Autodesk Fusion 360 part; units mm, degrees
(part 3 of 4)
sketch "Sketch3" plane through (0, 1.5, 0) normal (0, 1, 0) x (-1, 0, 0)
  arc A0 (-294.5875, 3) -> (-291.5875, 0) centre (-291.5875, 3) ccw
  line L0 (-291.5875, 0) -> (-3, 0)
  arc A1 (-3, 0) -> (0, 3) centre (-3, 3) ccw
  line L1 (0, 3) -> (0, 137)
  arc A2 (0, 137) -> (-3, 140) centre (-3, 137) ccw
  line L2 (-3, 140) -> (-327, 140)
  arc A3 (-327, 140) -> (-330, 137) centre (-327, 137) ccw
  line L3 (-330, 137) -> (-330, 70.475)
  arc A4 (-330, 70.475) -> (-327, 67.475) centre (-327, 70.475) ccw
  line L4 (-327, 67.475) -> (-297.5875, 67.475)
  arc A5 (-294.5875, 64.475) -> (-297.5875, 67.475) centre (-297.5875, 64.475) ccw
  line L5 (-294.5875, 64.475) -> (-294.5875, 3)
  arc A6 (-96.5875, 53.475) -> (-96.0875, 53.975) centre (-96.5875, 53.975) ccw
  line L6 (-96.5875, 53.475) -> (-109.5875, 53.475)
  arc A7 (-110.0875, 53.975) -> (-109.5875, 53.475) centre (-109.5875, 53.975) ccw
  line L7 (-110.0875, 53.975) -> (-110.0875, 66.975)
  arc A8 (-109.5875, 67.475) -> (-110.0875, 66.975) centre (-109.5875, 66.975) ccw
  line L8 (-109.5875, 67.475) -> (-96.5875, 67.475)
  arc A9 (-96.0875, 66.975) -> (-96.5875, 67.475) centre (-96.5875, 66.975) ccw
  line L9 (-96.0875, 66.975) -> (-96.0875, 53.975)
  line L10 (-105.6125, 24.1125) -> (-105.6125, 11.1125)
  arc A10 (-106.1125, 10.6125) -> (-105.6125, 11.1125) centre (-106.1125, 11.1125) ccw
  line L11 (-106.1125, 10.6125) -> (-119.1125, 10.6125)
  arc A11 (-119.6125, 11.1125) -> (-119.1125, 10.6125) centre (-119.1125, 11.1125) ccw
  line L12 (-119.6125, 11.1125) -> (-119.6125, 24.1125)
  arc A12 (-119.1125, 24.6125) -> (-119.6125, 24.1125) centre (-119.1125, 24.1125) ccw
  line L13 (-119.1125, 24.6125) -> (-106.1125, 24.6125)
  arc A13 (-105.6125, 24.1125) -> (-106.1125, 24.6125) centre (-106.1125, 24.1125) ccw
  arc A14 (-201.3625, 34.425) -> (-200.8625, 34.925) centre (-201.3625, 34.925) ccw
  line L14 (-201.3625, 34.425) -> (-214.3625, 34.425)
  arc A15 (-214.8625, 34.925) -> (-214.3625, 34.425) centre (-214.3625, 34.925) ccw
  line L15 (-214.8625, 34.925) -> (-214.8625, 47.925)
  arc A16 (-214.3625, 48.425) -> (-214.8625, 47.925) centre (-214.3625, 47.925) ccw
  line L16 (-214.3625, 48.425) -> (-201.3625, 48.425)
  arc A17 (-200.8625, 47.925) -> (-201.3625, 48.425) centre (-201.3625, 47.925) ccw
  line L17 (-200.8625, 47.925) -> (-200.8625, 34.925)
  arc A18 (-53.725, 91.575) -> (-53.225, 92.075) centre (-53.725, 92.075) ccw
  line L18 (-53.725, 91.575) -> (-66.725, 91.575)
  arc A19 (-67.225, 92.075) -> (-66.725, 91.575) centre (-66.725, 92.075) ccw
  line L19 (-67.225, 92.075) -> (-67.225, 105.075)
  arc A20 (-66.725, 105.575) -> (-67.225, 105.075) centre (-66.725, 105.075) ccw
  line L20 (-66.725, 105.575) -> (-53.725, 105.575)
  arc A21 (-53.225, 105.075) -> (-53.725, 105.575) centre (-53.725, 105.075) ccw
  line L21 (-53.225, 105.075) -> (-53.225, 92.075)
  arc A22 (-220.4125, 34.425) -> (-219.9125, 34.925) centre (-220.4125, 34.925) ccw
  line L22 (-220.4125, 34.425) -> (-233.4125, 34.425)
  arc A23 (-233.9125, 34.925) -> (-233.4125, 34.425) centre (-233.4125, 34.925) ccw
  line L23 (-233.9125, 34.925) -> (-233.9125, 47.925)
  arc A24 (-233.4125, 48.425) -> (-233.9125, 47.925) centre (-233.4125, 47.925) ccw
  line L24 (-233.4125, 48.425) -> (-220.4125, 48.425)
  arc A25 (-219.9125, 47.925) -> (-220.4125, 48.425) centre (-220.4125, 47.925) ccw
  line L25 (-219.9125, 47.925) -> (-219.9125, 34.925)
  arc A26 (-283.4755, 35.425) -> (-282.9755, 35.925) centre (-283.4755, 35.925) ccw
  line L26 (-283.4755, 35.425) -> (-289.4755, 35.425)
  arc A27 (-289.9755, 35.925) -> (-289.4755, 35.425) centre (-289.4755, 35.925) ccw
  line L27 (-289.9755, 35.925) -> (-289.9755, 49.925)
  arc A28 (-289.4755, 50.425) -> (-289.9755, 49.925) centre (-289.4755, 49.925) ccw
  line L28 (-289.4755, 50.425) -> (-283.4755, 50.425)
  arc A29 (-282.9755, 49.925) -> (-283.4755, 50.425) centre (-283.4755, 49.925) ccw
  line L29 (-282.9755, 49.925) -> (-282.9755, 35.925)
  arc A30 (-101.35, 72.525) -> (-100.85, 73.025) centre (-101.35, 73.025) ccw
  line L30 (-101.35, 72.525) -> (-114.35, 72.525)
  arc A31 (-114.85, 73.025) -> (-114.35, 72.525) centre (-114.35, 73.025) ccw
  line L31 (-114.85, 73.025) -> (-114.85, 86.025)
  arc A32 (-114.35, 86.525) -> (-114.85, 86.025) centre (-114.35, 86.025) ccw
  line L32 (-114.35, 86.525) -> (-101.35, 86.525)
  arc A33 (-100.85, 86.025) -> (-101.35, 86.525) centre (-101.35, 86.025) ccw
  line L33 (-100.85, 86.025) -> (-100.85, 73.025)
  arc A34 (-263.275, 115.3875) -> (-262.775, 115.8875) centre (-263.275, 115.8875) ccw
  line L34 (-263.275, 115.3875) -> (-276.275, 115.3875)
  arc A35 (-276.775, 115.8875) -> (-276.275, 115.3875) centre (-276.275, 115.8875) ccw
  line L35 (-276.775, 115.8875) -> (-276.775, 128.8875)
  arc A36 (-276.275, 129.3875) -> (-276.775, 128.8875) centre (-276.275, 128.8875) ccw
  line L36 (-276.275, 129.3875) -> (-263.275, 129.3875)
  arc A37 (-262.775, 128.8875) -> (-263.275, 129.3875) centre (-263.275, 128.8875) ccw
  line L37 (-262.775, 128.8875) -> (-262.775, 115.8875)
  arc A38 (-115.6375, 53.475) -> (-115.1375, 53.975) centre (-115.6375, 53.975) ccw
  line L38 (-115.6375, 53.475) -> (-128.6375, 53.475)
  arc A39 (-129.1375, 53.975) -> (-128.6375, 53.475) centre (-128.6375, 53.975) ccw
  line L39 (-129.1375, 53.975) -> (-129.1375, 66.975)
  arc A40 (-128.6375, 67.475) -> (-129.1375, 66.975) centre (-128.6375, 66.975) ccw
  line L40 (-128.6375, 67.475) -> (-115.6375, 67.475)
  arc A41 (-115.1375, 66.975) -> (-115.6375, 67.475) centre (-115.6375, 66.975) ccw
  line L41 (-115.1375, 66.975) -> (-115.1375, 53.975)
  line L42 (-36.5563, 124.125) -> (-36.5563, 111.125)
  arc A42 (-37.0563, 110.625) -> (-36.5563, 111.125) centre (-37.0563, 111.125) ccw
  line L43 (-37.0563, 110.625) -> (-50.0563, 110.625)
  arc A43 (-50.5563, 111.125) -> (-50.0563, 110.625) centre (-50.0563, 111.125) ccw
  line L44 (-50.5563, 111.125) -> (-50.5563, 124.125)
  arc A44 (-50.0563, 124.625) -> (-50.5563, 124.125) centre (-50.0563, 124.125) ccw
  line L45 (-50.0563, 124.625) -> (-37.0563, 124.625)
  arc A45 (-36.5563, 124.125) -> (-37.0563, 124.625) centre (-37.0563, 124.125) ccw
  arc A46 (-68.0125, 34.425) -> (-67.5125, 34.925) centre (-68.0125, 34.925) ccw
  line L46 (-68.0125, 34.425) -> (-81.0125, 34.425)
  arc A47 (-81.5125, 34.925) -> (-81.0125, 34.425) centre (-81.0125, 34.925) ccw
  line L47 (-81.5125, 34.925) -> (-81.5125, 47.925)
  arc A48 (-81.0125, 48.425) -> (-81.5125, 47.925) centre (-81.0125, 47.925) ccw
  line L48 (-81.0125, 48.425) -> (-68.0125, 48.425)
  arc A49 (-67.5125, 47.925) -> (-68.0125, 48.425) centre (-68.0125, 47.925) ccw
  line L49 (-67.5125, 47.925) -> (-67.5125, 34.925)
  arc A50 (-251.3688, 91.575) -> (-250.8688, 92.075) centre (-251.3688, 92.075) ccw
  line L50 (-251.3688, 91.575) -> (-264.3688, 91.575)
  arc A51 (-264.8688, 92.075) -> (-264.3688, 91.575) centre (-264.3688, 92.075) ccw
  line L51 (-264.8688, 92.075) -> (-264.8688, 105.075)
  arc A52 (-264.3688, 105.575) -> (-264.8688, 105.075) centre (-264.3688, 105.075) ccw
  line L52 (-264.3688, 105.575) -> (-251.3688, 105.575)
  arc A53 (-250.8688, 105.075) -> (-251.3688, 105.575) centre (-251.3688, 105.075) ccw
  line L53 (-250.8688, 105.075) -> (-250.8688, 92.075)
  arc A54 (-139.45, 72.525) -> (-138.95, 73.025) centre (-139.45, 73.025) ccw
  line L54 (-139.45, 72.525) -> (-152.45, 72.525)
  arc A55 (-152.95, 73.025) -> (-152.45, 72.525) centre (-152.45, 73.025) ccw
  line L55 (-152.95, 73.025) -> (-152.95, 86.025)
  arc A56 (-152.45, 86.525) -> (-152.95, 86.025) centre (-152.45, 86.025) ccw
  line L56 (-152.45, 86.525) -> (-139.45, 86.525)
  arc A57 (-138.95, 86.025) -> (-139.45, 86.525) centre (-139.45, 86.025) ccw
  line L57 (-138.95, 86.025) -> (-138.95, 73.025)
  arc A58 (-265.6563, 72.525) -> (-265.1563, 73.025) centre (-265.6563, 73.025) ccw
  line L58 (-265.6563, 72.525) -> (-278.6563, 72.525)
  arc A59 (-279.1563, 73.025) -> (-278.6563, 72.525) centre (-278.6563, 73.025) ccw
  line L59 (-279.1563, 73.025) -> (-279.1563, 86.025)
  arc A60 (-278.6563, 86.525) -> (-279.1563, 86.025) centre (-278.6563, 86.025) ccw
  line L60 (-278.6563, 86.525) -> (-265.6563, 86.525)
  arc A61 (-265.1563, 86.025) -> (-265.6563, 86.525) centre (-265.6563, 86.025) ccw
  line L61 (-265.1563, 86.025) -> (-265.1563, 73.025)
  line L62 (-110.375, 105.075) -> (-110.375, 92.075)
  arc A62 (-110.875, 91.575) -> (-110.375, 92.075) centre (-110.875, 92.075) ccw
  line L63 (-110.875, 91.575) -> (-123.875, 91.575)
  arc A63 (-124.375, 92.075) -> (-123.875, 91.575) centre (-123.875, 92.075) ccw
  line L64 (-124.375, 92.075) -> (-124.375, 105.075)
  arc A64 (-123.875, 105.575) -> (-124.375, 105.075) centre (-123.875, 105.075) ccw
  line L65 (-123.875, 105.575) -> (-110.875, 105.575)
  arc A65 (-110.375, 105.075) -> (-110.875, 105.575) centre (-110.875, 105.075) ccw
  arc A66 (-68.0125, 10.6125) -> (-67.5125, 11.1125) centre (-68.0125, 11.1125) ccw
  line L66 (-68.0125, 10.6125) -> (-81.0125, 10.6125)
  arc A67 (-81.5125, 11.1125) -> (-81.0125, 10.6125) centre (-81.0125, 11.1125) ccw
  line L67 (-81.5125, 11.1125) -> (-81.5125, 24.1125)
  arc A68 (-81.0125, 24.6125) -> (-81.5125, 24.1125) centre (-81.0125, 24.1125) ccw
  line L68 (-81.0125, 24.6125) -> (-68.0125, 24.6125)
  arc A69 (-67.5125, 24.1125) -> (-68.0125, 24.6125) centre (-68.0125, 24.1125) ccw
  line L69 (-67.5125, 24.1125) -> (-67.5125, 11.1125)
  arc A70 (-125.1625, 34.425) -> (-124.6625, 34.925) centre (-125.1625, 34.925) ccw
  line L70 (-125.1625, 34.425) -> (-138.1625, 34.425)
  arc A71 (-138.6625, 34.925) -> (-138.1625, 34.425) centre (-138.1625, 34.925) ccw
  line L71 (-138.6625, 34.925) -> (-138.6625, 47.925)
  arc A72 (-138.1625, 48.425) -> (-138.6625, 47.925) centre (-138.1625, 47.925) ccw
  line L72 (-138.1625, 48.425) -> (-125.1625, 48.425)
  arc A73 (-124.6625, 47.925) -> (-125.1625, 48.425) centre (-125.1625, 47.925) ccw
  line L73 (-124.6625, 47.925) -> (-124.6625, 34.925)
  line L74 (-43.7, 86.025) -> (-43.7, 73.025)
  arc A74 (-44.2, 72.525) -> (-43.7, 73.025) centre (-44.2, 73.025) ccw
  line L75 (-44.2, 72.525) -> (-57.2, 72.525)
  arc A75 (-57.7, 73.025) -> (-57.2, 72.525) centre (-57.2, 73.025) ccw
  line L76 (-57.7, 73.025) -> (-57.7, 86.025)
  arc A76 (-57.2, 86.525) -> (-57.7, 86.025) centre (-57.2, 86.025) ccw
  line L77 (-57.2, 86.525) -> (-44.2, 86.525)
  arc A77 (-43.7, 86.025) -> (-44.2, 86.525) centre (-44.2, 86.025) ccw
  arc A78 (-220.4125, 10.6125) -> (-219.9125, 11.1125) centre (-220.4125, 11.1125) ccw
  line L78 (-220.4125, 10.6125) -> (-233.4125, 10.6125)
  arc A79 (-233.9125, 11.1125) -> (-233.4125, 10.6125) centre (-233.4125, 11.1125) ccw
  line L79 (-233.9125, 11.1125) -> (-233.9125, 24.1125)
  arc A80 (-233.4125, 24.6125) -> (-233.9125, 24.1125) centre (-233.4125, 24.1125) ccw
  line L80 (-233.4125, 24.6125) -> (-220.4125, 24.6125)
  arc A81 (-219.9125, 24.1125) -> (-220.4125, 24.6125) centre (-220.4125, 24.1125) ccw
  line L81 (-219.9125, 24.1125) -> (-219.9125, 11.1125)
  arc A82 (-201.3625, 110.625) -> (-200.8625, 111.125) centre (-201.3625, 111.125) ccw
  line L82 (-201.3625, 110.625) -> (-214.3625, 110.625)
  arc A83 (-214.8625, 111.125) -> (-214.3625, 110.625) centre (-214.3625, 111.125) ccw
  line L83 (-214.8625, 111.125) -> (-214.8625, 124.125)
  arc A84 (-214.3625, 124.625) -> (-214.8625, 124.125) centre (-214.3625, 124.125) ccw
  line L84 (-214.3625, 124.625) -> (-201.3625, 124.625)
  arc A85 (-200.8625, 124.125) -> (-201.3625, 124.625) centre (-201.3625, 124.125) ccw
  line L85 (-200.8625, 124.125) -> (-200.8625, 111.125)
  arc A86 (-257.2183, 73.525) -> (-256.7183, 74.025) centre (-257.2183, 74.025) ccw
  line L86 (-257.2183, 73.525) -> (-263.2183, 73.525)
  arc A87 (-263.7183, 74.025) -> (-263.2183, 73.525) centre (-263.2183, 74.025) ccw
  line L87 (-263.7183, 74.025) -> (-263.7183, 88.025)
  arc A88 (-263.2183, 88.525) -> (-263.7183, 88.025) centre (-263.2183, 88.025) ccw
  line L88 (-263.2183, 88.525) -> (-257.2183, 88.525)
  arc A89 (-256.7183, 88.025) -> (-257.2183, 88.525) centre (-257.2183, 88.025) ccw
  line L89 (-256.7183, 88.025) -> (-256.7183, 74.025)
  arc A90 (-177.55, 72.525) -> (-177.05, 73.025) centre (-177.55, 73.025) ccw
  line L90 (-177.55, 72.525) -> (-190.55, 72.525)
  arc A91 (-191.05, 73.025) -> (-190.55, 72.525) centre (-190.55, 73.025) ccw
  line L91 (-191.05, 73.025) -> (-191.05, 86.025)
  arc A92 (-190.55, 86.525) -> (-191.05, 86.025) centre (-190.55, 86.025) ccw
  line L92 (-190.55, 86.525) -> (-177.55, 86.525)
  arc A93 (-177.05, 86.025) -> (-177.55, 86.525) centre (-177.55, 86.025) ccw
  line L93 (-177.05, 86.025) -> (-177.05, 73.025)
  arc A94 (-158.5, 72.525) -> (-158, 73.025) centre (-158.5, 73.025) ccw
  line L94 (-158.5, 72.525) -> (-171.5, 72.525)
  arc A95 (-172, 73.025) -> (-171.5, 72.525) centre (-171.5, 73.025) ccw
  line L95 (-172, 73.025) -> (-172, 86.025)
  arc A96 (-171.5, 86.525) -> (-172, 86.025) centre (-171.5, 86.025) ccw
  line L96 (-171.5, 86.525) -> (-158.5, 86.525)
  arc A97 (-158, 86.025) -> (-158.5, 86.525) centre (-158.5, 86.025) ccw
  line L97 (-158, 86.025) -> (-158, 73.025)
  arc A98 (-234.7, 72.525) -> (-234.2, 73.025) centre (-234.7, 73.025) ccw
  line L98 (-234.7, 72.525) -> (-247.7, 72.525)
  arc A99 (-248.2, 73.025) -> (-247.7, 72.525) centre (-247.7, 73.025) ccw
  line L99 (-248.2, 73.025) -> (-248.2, 86.025)
  arc A100 (-247.7, 86.525) -> (-248.2, 86.025) centre (-247.7, 86.025) ccw
  line L100 (-247.7, 86.525) -> (-234.7, 86.525)
  arc A101 (-234.2, 86.025) -> (-234.7, 86.525) centre (-234.7, 86.025) ccw
  line L101 (-234.2, 86.025) -> (-234.2, 73.025)
  arc A102 (-215.65, 72.525) -> (-215.15, 73.025) centre (-215.65, 73.025) ccw
  line L102 (-215.65, 72.525) -> (-228.65, 72.525)
  arc A103 (-229.15, 73.025) -> (-228.65, 72.525) centre (-228.65, 73.025) ccw
  line L103 (-229.15, 73.025) -> (-229.15, 86.025)
  arc A104 (-228.65, 86.525) -> (-229.15, 86.025) centre (-228.65, 86.025) ccw
  line L104 (-228.65, 86.525) -> (-215.65, 86.525)
  arc A105 (-215.15, 86.025) -> (-215.65, 86.525) centre (-215.65, 86.025) ccw
  line L105 (-215.15, 86.025) -> (-215.15, 73.025)
  arc A106 (-210.8875, 53.475) -> (-210.3875, 53.975) centre (-210.8875, 53.975) ccw
  line L106 (-210.8875, 53.475) -> (-223.8875, 53.475)
  arc A107 (-224.3875, 53.975) -> (-223.8875, 53.475) centre (-223.8875, 53.975) ccw
  line L107 (-224.3875, 53.975) -> (-224.3875, 66.975)
  arc A108 (-223.8875, 67.475) -> (-224.3875, 66.975) centre (-223.8875, 66.975) ccw
  line L108 (-223.8875, 67.475) -> (-210.8875, 67.475)
  arc A109 (-210.3875, 66.975) -> (-210.8875, 67.475) centre (-210.8875, 66.975) ccw
  line L109 (-210.3875, 66.975) -> (-210.3875, 53.975)
  arc A110 (-191.8375, 53.475) -> (-191.3375, 53.975) centre (-191.8375, 53.975) ccw
  line L110 (-191.8375, 53.475) -> (-204.8375, 53.475)
  arc A111 (-205.3375, 53.975) -> (-204.8375, 53.475) centre (-204.8375, 53.975) ccw
  line L111 (-205.3375, 53.975) -> (-205.3375, 66.975)
  arc A112 (-204.8375, 67.475) -> (-205.3375, 66.975) centre (-204.8375, 66.975) ccw
  line L112 (-204.8375, 67.475) -> (-191.8375, 67.475)
  arc A113 (-191.3375, 66.975) -> (-191.8375, 67.475) centre (-191.8375, 66.975) ccw
  line L113 (-191.3375, 66.975) -> (-191.3375, 53.975)
  arc A114 (-196.6, 72.525) -> (-196.1, 73.025) centre (-196.6, 73.025) ccw
  line L114 (-196.6, 72.525) -> (-209.6, 72.525)
  arc A115 (-210.1, 73.025) -> (-209.6, 72.525) centre (-209.6, 73.025) ccw
  line L115 (-210.1, 73.025) -> (-210.1, 86.025)
  arc A116 (-209.6, 86.525) -> (-210.1, 86.025) centre (-209.6, 86.025) ccw
  line L116 (-209.6, 86.525) -> (-196.6, 86.525)
  arc A117 (-196.1, 86.025) -> (-196.6, 86.525) centre (-196.6, 86.025) ccw
  line L117 (-196.1, 86.025) -> (-196.1, 73.025)
  arc A118 (-172.7875, 53.475) -> (-172.2875, 53.975) centre (-172.7875, 53.975) ccw
  line L118 (-172.7875, 53.475) -> (-185.7875, 53.475)
  arc A119 (-186.2875, 53.975) -> (-185.7875, 53.475) centre (-185.7875, 53.975) ccw
  line L119 (-186.2875, 53.975) -> (-186.2875, 66.975)
  arc A120 (-185.7875, 67.475) -> (-186.2875, 66.975) centre (-185.7875, 66.975) ccw
  line L120 (-185.7875, 67.475) -> (-172.7875, 67.475)
  arc A121 (-172.2875, 66.975) -> (-172.7875, 67.475) centre (-172.7875, 66.975) ccw
  line L121 (-172.2875, 66.975) -> (-172.2875, 53.975)
  arc A122 (-181.525, 92.075) -> (-181.025, 91.575) centre (-181.025, 92.075) ccw
  line L122 (-181.525, 92.075) -> (-181.525, 105.075)
  arc A123 (-181.025, 105.575) -> (-181.525, 105.075) centre (-181.025, 105.075) ccw
  line L123 (-181.025, 105.575) -> (-168.025, 105.575)
  arc A124 (-167.525, 105.075) -> (-168.025, 105.575) centre (-168.025, 105.075) ccw
  line L124 (-167.525, 105.075) -> (-167.525, 92.075)
  arc A125 (-168.025, 91.575) -> (-167.525, 92.075) centre (-168.025, 92.075) ccw
  line L125 (-168.025, 91.575) -> (-181.025, 91.575)
  arc A126 (-200.575, 92.075) -> (-200.075, 91.575) centre (-200.075, 92.075) ccw
  line L126 (-200.575, 92.075) -> (-200.575, 105.075)
  arc A127 (-200.075, 105.575) -> (-200.575, 105.075) centre (-200.075, 105.075) ccw
  line L127 (-200.075, 105.575) -> (-187.075, 105.575)
  arc A128 (-186.575, 105.075) -> (-187.075, 105.575) centre (-187.075, 105.075) ccw
  line L128 (-186.575, 105.075) -> (-186.575, 92.075)
  arc A129 (-187.075, 91.575) -> (-186.575, 92.075) centre (-187.075, 92.075) ccw
  line L129 (-187.075, 91.575) -> (-200.075, 91.575)
  arc A130 (-182.3125, 34.425) -> (-181.8125, 34.925) centre (-182.3125, 34.925) ccw
  line L130 (-182.3125, 34.425) -> (-195.3125, 34.425)
  arc A131 (-195.8125, 34.925) -> (-195.3125, 34.425) centre (-195.3125, 34.925) ccw
  line L131 (-195.8125, 34.925) -> (-195.8125, 47.925)
  arc A132 (-195.3125, 48.425) -> (-195.8125, 47.925) centre (-195.3125, 47.925) ccw
  line L132 (-195.3125, 48.425) -> (-182.3125, 48.425)
  arc A133 (-181.8125, 47.925) -> (-182.3125, 48.425) centre (-182.3125, 47.925) ccw
  line L133 (-181.8125, 47.925) -> (-181.8125, 34.925)
  line L134 (-162.7625, 24.1125) -> (-162.7625, 11.1125)
  arc A134 (-163.2625, 10.6125) -> (-162.7625, 11.1125) centre (-163.2625, 11.1125) ccw
  line L135 (-163.2625, 10.6125) -> (-176.2625, 10.6125)
  arc A135 (-176.7625, 11.1125) -> (-176.2625, 10.6125) centre (-176.2625, 11.1125) ccw
  line L136 (-176.7625, 11.1125) -> (-176.7625, 24.1125)
  arc A136 (-176.2625, 24.6125) -> (-176.7625, 24.1125) centre (-176.2625, 24.1125) ccw
  line L137 (-176.2625, 24.6125) -> (-163.2625, 24.6125)
  arc A137 (-162.7625, 24.1125) -> (-163.2625, 24.6125) centre (-163.2625, 24.1125) ccw
  line L138 (-229.4375, 66.975) -> (-229.4375, 53.975)
  arc A138 (-229.9375, 53.475) -> (-229.4375, 53.975) centre (-229.9375, 53.975) ccw
  line L139 (-229.9375, 53.475) -> (-242.9375, 53.475)
  arc A139 (-243.4375, 53.975) -> (-242.9375, 53.475) centre (-242.9375, 53.975) ccw
  line L140 (-243.4375, 53.975) -> (-243.4375, 66.975)
  arc A140 (-242.9375, 67.475) -> (-243.4375, 66.975) centre (-242.9375, 66.975) ccw
  line L141 (-242.9375, 67.475) -> (-229.9375, 67.475)
  arc A141 (-229.4375, 66.975) -> (-229.9375, 67.475) centre (-229.9375, 66.975) ccw
  line L142 (-77.0375, 66.975) -> (-77.0375, 53.975)
  arc A142 (-77.5375, 53.475) -> (-77.0375, 53.975) centre (-77.5375, 53.975) ccw
  line L143 (-77.5375, 53.475) -> (-90.5375, 53.475)
  arc A143 (-91.0375, 53.975) -> (-90.5375, 53.475) centre (-90.5375, 53.975) ccw
  line L144 (-91.0375, 53.975) -> (-91.0375, 66.975)
  arc A144 (-90.5375, 67.475) -> (-91.0375, 66.975) centre (-90.5375, 66.975) ccw
  line L145 (-90.5375, 67.475) -> (-77.5375, 67.475)
  arc A145 (-77.0375, 66.975) -> (-77.5375, 67.475) centre (-77.5375, 66.975) ccw
  arc A146 (-225.175, 91.575) -> (-224.675, 92.075) centre (-225.175, 92.075) ccw
  line L146 (-225.175, 91.575) -> (-238.175, 91.575)
  arc A147 (-238.675, 92.075) -> (-238.175, 91.575) centre (-238.175, 92.075) ccw
  line L147 (-238.675, 92.075) -> (-238.675, 105.075)
  arc A148 (-238.175, 105.575) -> (-238.675, 105.075) centre (-238.175, 105.075) ccw
  line L148 (-238.175, 105.575) -> (-225.175, 105.575)
  arc A149 (-224.675, 105.075) -> (-225.175, 105.575) centre (-225.175, 105.075) ccw
  line L149 (-224.675, 105.075) -> (-224.675, 92.075)
  arc A150 (-153.7375, 53.475) -> (-153.2375, 53.975) centre (-153.7375, 53.975) ccw
  line L150 (-153.7375, 53.475) -> (-166.7375, 53.475)
  arc A151 (-167.2375, 53.975) -> (-166.7375, 53.475) centre (-166.7375, 53.975) ccw
  line L151 (-167.2375, 53.975) -> (-167.2375, 66.975)
  arc A152 (-166.7375, 67.475) -> (-167.2375, 66.975) centre (-166.7375, 66.975) ccw
  line L152 (-166.7375, 67.475) -> (-153.7375, 67.475)
  arc A153 (-153.2375, 66.975) -> (-153.7375, 67.475) centre (-153.7375, 66.975) ccw
  line L153 (-153.2375, 66.975) -> (-153.2375, 53.975)
  arc A154 (-163.2625, 34.425) -> (-162.7625, 34.925) centre (-163.2625, 34.925) ccw
  line L154 (-163.2625, 34.425) -> (-176.2625, 34.425)
  arc A155 (-176.7625, 34.925) -> (-176.2625, 34.425) centre (-176.2625, 34.925) ccw
  line L155 (-176.7625, 34.925) -> (-176.7625, 47.925)
  arc A156 (-176.2625, 48.425) -> (-176.7625, 47.925) centre (-176.2625, 47.925) ccw
  line L156 (-176.2625, 48.425) -> (-163.2625, 48.425)
  arc A157 (-162.7625, 47.925) -> (-163.2625, 48.425) centre (-163.2625, 47.925) ccw
  line L157 (-162.7625, 47.925) -> (-162.7625, 34.925)
  arc A158 (-148.975, 91.575) -> (-148.475, 92.075) centre (-148.975, 92.075) ccw
  line L158 (-148.975, 91.575) -> (-161.975, 91.575)
  arc A159 (-162.475, 92.075) -> (-161.975, 91.575) centre (-161.975, 92.075) ccw
  line L159 (-162.475, 92.075) -> (-162.475, 105.075)
  arc A160 (-161.975, 105.575) -> (-162.475, 105.075) centre (-161.975, 105.075) ccw
  line L160 (-161.975, 105.575) -> (-148.975, 105.575)
  arc A161 (-148.475, 105.075) -> (-148.975, 105.575) centre (-148.975, 105.075) ccw
  line L161 (-148.475, 105.075) -> (-148.475, 92.075)
  arc A162 (-195.8125, 11.1125) -> (-195.3125, 10.6125) centre (-195.3125, 11.1125) ccw
  line L162 (-195.8125, 11.1125) -> (-195.8125, 24.1125)
  arc A163 (-195.3125, 24.6125) -> (-195.8125, 24.1125) centre (-195.3125, 24.1125) ccw
  line L163 (-195.3125, 24.6125) -> (-182.3125, 24.6125)
  arc A164 (-181.8125, 24.1125) -> (-182.3125, 24.6125) centre (-182.3125, 24.1125) ccw
  line L164 (-181.8125, 24.1125) -> (-181.8125, 11.1125)
  arc A165 (-182.3125, 10.6125) -> (-181.8125, 11.1125) centre (-182.3125, 11.1125) ccw
  line L165 (-182.3125, 10.6125) -> (-195.3125, 10.6125)
  line L166 (-72.275, 105.075) -> (-72.275, 92.075)
  arc A166 (-72.775, 91.575) -> (-72.275, 92.075) centre (-72.775, 92.075) ccw
  line L167 (-72.775, 91.575) -> (-85.775, 91.575)
  arc A167 (-86.275, 92.075) -> (-85.775, 91.575) centre (-85.775, 92.075) ccw
  line L168 (-86.275, 92.075) -> (-86.275, 105.075)
  arc A168 (-85.775, 105.575) -> (-86.275, 105.075) centre (-85.775, 105.075) ccw
  line L169 (-85.775, 105.575) -> (-72.775, 105.575)
  arc A169 (-72.275, 105.075) -> (-72.775, 105.575) centre (-72.775, 105.075) ccw
  line L170 (-81.8, 86.025) -> (-81.8, 73.025)
  arc A170 (-82.3, 72.525) -> (-81.8, 73.025) centre (-82.3, 73.025) ccw
  line L171 (-82.3, 72.525) -> (-95.3, 72.525)
  arc A171 (-95.8, 73.025) -> (-95.3, 72.525) centre (-95.3, 73.025) ccw
  line L172 (-95.8, 73.025) -> (-95.8, 86.025)
  arc A172 (-95.3, 86.525) -> (-95.8, 86.025) centre (-95.3, 86.025) ccw
  line L173 (-95.3, 86.525) -> (-82.3, 86.525)
  arc A173 (-81.8, 86.025) -> (-82.3, 86.525) centre (-82.3, 86.025) ccw
  arc A174 (-248.9875, 53.475) -> (-248.4875, 53.975) centre (-248.9875, 53.975) ccw
  line L174 (-248.9875, 53.475) -> (-261.9875, 53.475)
  arc A175 (-262.4875, 53.975) -> (-261.9875, 53.475) centre (-261.9875, 53.975) ccw
  line L175 (-262.4875, 53.975) -> (-262.4875, 66.975)
  arc A176 (-261.9875, 67.475) -> (-262.4875, 66.975) centre (-261.9875, 66.975) ccw
  line L176 (-261.9875, 67.475) -> (-248.9875, 67.475)
  arc A177 (-248.4875, 66.975) -> (-248.9875, 67.475) centre (-248.9875, 66.975) ccw
  line L177 (-248.4875, 66.975) -> (-248.4875, 53.975)
  arc A178 (-272.8, 53.475) -> (-272.3, 53.975) centre (-272.8, 53.975) ccw
  line L178 (-272.8, 53.475) -> (-285.8, 53.475)
  arc A179 (-286.3, 53.975) -> (-285.8, 53.475) centre (-285.8, 53.975) ccw
  line L179 (-286.3, 53.975) -> (-286.3, 66.975)
  arc A180 (-285.8, 67.475) -> (-286.3, 66.975) centre (-285.8, 66.975) ccw
  line L180 (-285.8, 67.475) -> (-272.8, 67.475)
  arc A181 (-272.3, 66.975) -> (-272.8, 67.475) centre (-272.8, 66.975) ccw
  line L181 (-272.3, 66.975) -> (-272.3, 53.975)
  line L182 (-185.3063, 126.125) -> (-185.3063, 112.125)
  arc A182 (-185.8063, 111.625) -> (-185.3063, 112.125) centre (-185.8063, 112.125) ccw
  line L183 (-185.8063, 111.625) -> (-191.8063, 111.625)
  arc A183 (-192.3063, 112.125) -> (-191.8063, 111.625) centre (-191.8063, 112.125) ccw
  line L184 (-192.3063, 112.125) -> (-192.3063, 126.125)
  arc A184 (-191.8063, 126.625) -> (-192.3063, 126.125) centre (-191.8063, 126.125) ccw
  line L185 (-191.8063, 126.625) -> (-185.8063, 126.625)
  arc A185 (-185.3063, 126.125) -> (-185.8063, 126.625) centre (-185.8063, 126.125) ccw
  line L186 (-205.625, 105.075) -> (-205.625, 92.075)
  arc A186 (-206.125, 91.575) -> (-205.625, 92.075) centre (-206.125, 92.075) ccw
  line L187 (-206.125, 91.575) -> (-219.125, 91.575)
  arc A187 (-219.625, 92.075) -> (-219.125, 91.575) centre (-219.125, 92.075) ccw
  line L188 (-219.625, 92.075) -> (-219.625, 105.075)
  arc A188 (-219.125, 105.575) -> (-219.625, 105.075) centre (-219.125, 105.075) ccw
  line L189 (-219.125, 105.575) -> (-206.125, 105.575)
  arc A189 (-205.625, 105.075) -> (-206.125, 105.575) centre (-206.125, 105.075) ccw
  arc A190 (-259.5995, 35.425) -> (-259.0995, 35.925) centre (-259.5995, 35.925) ccw
  line L190 (-259.5995, 35.425) -> (-265.5995, 35.425)
  arc A191 (-266.0995, 35.925) -> (-265.5995, 35.425) centre (-265.5995, 35.925) ccw
  line L191 (-266.0995, 35.925) -> (-266.0995, 49.925)
  arc A192 (-265.5995, 50.425) -> (-266.0995, 49.925) centre (-265.5995, 49.925) ccw
  line L192 (-265.5995, 50.425) -> (-259.5995, 50.425)
  arc A193 (-259.0995, 49.925) -> (-259.5995, 50.425) centre (-259.5995, 49.925) ccw
  line L193 (-259.0995, 49.925) -> (-259.0995, 35.925)
  arc A194 (-252.9625, 34.925) -> (-252.4625, 34.425) centre (-252.4625, 34.925) ccw
  line L194 (-252.9625, 34.925) -> (-252.9625, 47.925)
  arc A195 (-252.4625, 48.425) -> (-252.9625, 47.925) centre (-252.4625, 47.925) ccw
  line L195 (-252.4625, 48.425) -> (-239.4625, 48.425)
  arc A196 (-238.9625, 47.925) -> (-239.4625, 48.425) centre (-239.4625, 47.925) ccw
  line L196 (-238.9625, 47.925) -> (-238.9625, 34.925)
  arc A197 (-239.4625, 34.425) -> (-238.9625, 34.925) centre (-239.4625, 34.925) ccw
  line L197 (-239.4625, 34.425) -> (-252.4625, 34.425)
  arc A198 (-63.25, 72.525) -> (-62.75, 73.025) centre (-63.25, 73.025) ccw
  line L198 (-63.25, 72.525) -> (-76.25, 72.525)
  arc A199 (-76.75, 73.025) -> (-76.25, 72.525) centre (-76.25, 73.025) ccw
  line L199 (-76.75, 73.025) -> (-76.75, 86.025)
  arc A200 (-76.25, 86.525) -> (-76.75, 86.025) centre (-76.25, 86.025) ccw
  line L200 (-76.25, 86.525) -> (-63.25, 86.525)
  arc A201 (-62.75, 86.025) -> (-63.25, 86.525) centre (-63.25, 86.025) ccw
  line L201 (-62.75, 86.025) -> (-62.75, 73.025)
  arc A202 (-144.2125, 34.425) -> (-143.7125, 34.925) centre (-144.2125, 34.925) ccw
  line L202 (-144.2125, 34.425) -> (-157.2125, 34.425)
  arc A203 (-157.7125, 34.925) -> (-157.2125, 34.425) centre (-157.2125, 34.925) ccw
  line L203 (-157.7125, 34.925) -> (-157.7125, 47.925)
  arc A204 (-157.2125, 48.425) -> (-157.7125, 47.925) centre (-157.2125, 47.925) ccw
  line L204 (-157.2125, 48.425) -> (-144.2125, 48.425)
  arc A205 (-143.7125, 47.925) -> (-144.2125, 48.425) centre (-144.2125, 47.925) ccw
  line L205 (-143.7125, 47.925) -> (-143.7125, 34.925)
  arc A206 (-272.0125, 11.1125) -> (-271.5125, 10.6125) centre (-271.5125, 11.1125) ccw
  line L206 (-272.0125, 11.1125) -> (-272.0125, 24.1125)
  arc A207 (-271.5125, 24.6125) -> (-272.0125, 24.1125) centre (-271.5125, 24.1125) ccw
  line L207 (-271.5125, 24.6125) -> (-258.5125, 24.6125)
  arc A208 (-258.0125, 24.1125) -> (-258.5125, 24.6125) centre (-258.5125, 24.1125) ccw
  line L208 (-258.0125, 24.1125) -> (-258.0125, 11.1125)
  arc A209 (-258.5125, 10.6125) -> (-258.0125, 11.1125) centre (-258.5125, 11.1125) ccw
  line L209 (-258.5125, 10.6125) -> (-271.5125, 10.6125)
  arc A210 (-71.9875, 53.975) -> (-71.4875, 53.475) centre (-71.4875, 53.975) ccw
  line L210 (-71.9875, 53.975) -> (-71.9875, 66.975)
  arc A211 (-71.4875, 67.475) -> (-71.9875, 66.975) centre (-71.4875, 66.975) ccw
  line L211 (-71.4875, 67.475) -> (-58.4875, 67.475)
  arc A212 (-57.9875, 66.975) -> (-58.4875, 67.475) centre (-58.4875, 66.975) ccw
  line L212 (-57.9875, 66.975) -> (-57.9875, 53.975)
  arc A213 (-58.4875, 53.475) -> (-57.9875, 53.975) centre (-58.4875, 53.975) ccw
  line L213 (-58.4875, 53.475) -> (-71.4875, 53.475)
  arc A214 (-39.4375, 53.475) -> (-38.9375, 53.975) centre (-39.4375, 53.975) ccw
  line L214 (-39.4375, 53.475) -> (-52.4375, 53.475)
  arc A215 (-52.9375, 53.975) -> (-52.4375, 53.475) centre (-52.4375, 53.975) ccw
  line L215 (-52.9375, 53.975) -> (-52.9375, 66.975)
  arc A216 (-52.4375, 67.475) -> (-52.9375, 66.975) centre (-52.4375, 66.975) ccw
  line L216 (-52.4375, 67.475) -> (-39.4375, 67.475)
  arc A217 (-38.9375, 66.975) -> (-39.4375, 67.475) centre (-39.4375, 66.975) ccw
  line L217 (-38.9375, 66.975) -> (-38.9375, 53.975)
  arc A218 (-48.9625, 10.6125) -> (-48.4625, 11.1125) centre (-48.9625, 11.1125) ccw
  line L218 (-48.9625, 10.6125) -> (-61.9625, 10.6125)
  arc A219 (-62.4625, 11.1125) -> (-61.9625, 10.6125) centre (-61.9625, 11.1125) ccw
  line L219 (-62.4625, 11.1125) -> (-62.4625, 24.1125)
  arc A220 (-61.9625, 24.6125) -> (-62.4625, 24.1125) centre (-61.9625, 24.1125) ccw
  line L220 (-61.9625, 24.6125) -> (-48.9625, 24.6125)
  arc A221 (-48.4625, 24.1125) -> (-48.9625, 24.6125) centre (-48.9625, 24.1125) ccw
  line L221 (-48.4625, 24.1125) -> (-48.4625, 11.1125)
  arc A222 (-239.4625, 10.6125) -> (-238.9625, 11.1125) centre (-239.4625, 11.1125) ccw
  line L222 (-239.4625, 10.6125) -> (-252.4625, 10.6125)
  arc A223 (-252.9625, 11.1125) -> (-252.4625, 10.6125) centre (-252.4625, 11.1125) ccw
  line L223 (-252.9625, 11.1125) -> (-252.9625, 24.1125)
  arc A224 (-252.4625, 24.6125) -> (-252.9625, 24.1125) centre (-252.4625, 24.1125) ccw
  line L224 (-252.4625, 24.6125) -> (-239.4625, 24.6125)
  arc A225 (-238.9625, 24.1125) -> (-239.4625, 24.6125) centre (-239.4625, 24.1125) ccw
  line L225 (-238.9625, 24.1125) -> (-238.9625, 11.1125)
  arc A226 (-106.1125, 34.425) -> (-105.6125, 34.925) centre (-106.1125, 34.925) ccw
  line L226 (-106.1125, 34.425) -> (-119.1125, 34.425)
  arc A227 (-119.6125, 34.925) -> (-119.1125, 34.425) centre (-119.1125, 34.925) ccw
  line L227 (-119.6125, 34.925) -> (-119.6125, 47.925)
  arc A228 (-119.1125, 48.425) -> (-119.6125, 47.925) centre (-119.1125, 47.925) ccw
  line L228 (-119.1125, 48.425) -> (-106.1125, 48.425)
  arc A229 (-105.6125, 47.925) -> (-106.1125, 48.425) centre (-106.1125, 47.925) ccw
  line L229 (-105.6125, 47.925) -> (-105.6125, 34.925)
  arc A230 (-18.0063, 72.525) -> (-17.5063, 73.025) centre (-18.0063, 73.025) ccw
  line L230 (-18.0063, 72.525) -> (-31.0063, 72.525)
  arc A231 (-31.5063, 73.025) -> (-31.0063, 72.525) centre (-31.0063, 73.025) ccw
  line L231 (-31.5063, 73.025) -> (-31.5063, 86.025)
  arc A232 (-31.0063, 86.525) -> (-31.5063, 86.025) centre (-31.0063, 86.025) ccw
  line L232 (-31.0063, 86.525) -> (-18.0063, 86.525)
  arc A233 (-17.5063, 86.025) -> (-18.0063, 86.525) centre (-18.0063, 86.025) ccw
  line L233 (-17.5063, 86.025) -> (-17.5063, 73.025)
  line L234 (-10.3625, 47.925) -> (-10.3625, 34.925)
  arc A234 (-10.8625, 34.425) -> (-10.3625, 34.925) centre (-10.8625, 34.925) ccw
  line L235 (-10.8625, 34.425) -> (-23.8625, 34.425)
  arc A235 (-24.3625, 34.925) -> (-23.8625, 34.425) centre (-23.8625, 34.925) ccw
  line L236 (-24.3625, 34.925) -> (-24.3625, 47.925)
  arc A236 (-23.8625, 48.425) -> (-24.3625, 47.925) centre (-23.8625, 47.925) ccw
  line L237 (-23.8625, 48.425) -> (-10.8625, 48.425)
  arc A237 (-10.3625, 47.925) -> (-10.8625, 48.425) centre (-10.8625, 47.925) ccw
  arc A238 (-277.5625, 10.6125) -> (-277.0625, 11.1125) centre (-277.5625, 11.1125) ccw
  line L238 (-277.5625, 10.6125) -> (-290.5625, 10.6125)
  arc A239 (-291.0625, 11.1125) -> (-290.5625, 10.6125) centre (-290.5625, 11.1125) ccw
  line L239 (-291.0625, 11.1125) -> (-291.0625, 24.1125)
  arc A240 (-290.5625, 24.6125) -> (-291.0625, 24.1125) centre (-290.5625, 24.1125) ccw
  line L240 (-290.5625, 24.6125) -> (-277.5625, 24.6125)
  arc A241 (-277.0625, 24.1125) -> (-277.5625, 24.6125) centre (-277.5625, 24.1125) ccw
  line L241 (-277.0625, 24.1125) -> (-277.0625, 11.1125)
  arc A242 (-125.1625, 10.6125) -> (-124.6625, 11.1125) centre (-125.1625, 11.1125) ccw
  line L242 (-125.1625, 10.6125) -> (-138.1625, 10.6125)
  arc A243 (-138.6625, 11.1125) -> (-138.1625, 10.6125) centre (-138.1625, 11.1125) ccw
  line L243 (-138.6625, 11.1125) -> (-138.6625, 24.1125)
  arc A244 (-138.1625, 24.6125) -> (-138.6625, 24.1125) centre (-138.1625, 24.1125) ccw
  line L244 (-138.1625, 24.6125) -> (-125.1625, 24.6125)
  arc A245 (-124.6625, 24.1125) -> (-125.1625, 24.6125) centre (-125.1625, 24.1125) ccw
  line L245 (-124.6625, 24.1125) -> (-124.6625, 11.1125)
  arc A246 (-48.9625, 34.425) -> (-48.4625, 34.925) centre (-48.9625, 34.925) ccw
  line L246 (-48.9625, 34.425) -> (-61.9625, 34.425)
  arc A247 (-62.4625, 34.925) -> (-61.9625, 34.425) centre (-61.9625, 34.925) ccw
  line L247 (-62.4625, 34.925) -> (-62.4625, 47.925)
  arc A248 (-61.9625, 48.425) -> (-62.4625, 47.925) centre (-61.9625, 47.925) ccw
  line L248 (-61.9625, 48.425) -> (-48.9625, 48.425)
  arc A249 (-48.4625, 47.925) -> (-48.9625, 48.425) centre (-48.9625, 47.925) ccw
  line L249 (-48.4625, 47.925) -> (-48.4625, 34.925)
  arc A250 (-220.4125, 110.625) -> (-219.9125, 111.125) centre (-220.4125, 111.125) ccw
  line L250 (-220.4125, 110.625) -> (-233.4125, 110.625)
  arc A251 (-233.9125, 111.125) -> (-233.4125, 110.625) centre (-233.4125, 111.125) ccw
  line L251 (-233.9125, 111.125) -> (-233.9125, 124.125)
  arc A252 (-233.4125, 124.625) -> (-233.9125, 124.125) centre (-233.4125, 124.125) ccw
  line L252 (-233.4125, 124.625) -> (-220.4125, 124.625)
  arc A253 (-219.9125, 124.125) -> (-220.4125, 124.625) centre (-220.4125, 124.125) ccw
  line L253 (-219.9125, 124.125) -> (-219.9125, 111.125)
  arc A254 (-38.2068, 92.575) -> (-37.7068, 93.075) centre (-38.2068, 93.075) ccw
  line L254 (-38.2068, 92.575) -> (-44.2068, 92.575)
  arc A255 (-44.7068, 93.075) -> (-44.2068, 92.575) centre (-44.2068, 93.075) ccw
  line L255 (-44.7068, 93.075) -> (-44.7068, 107.075)
  arc A256 (-44.2068, 107.575) -> (-44.7068, 107.075) centre (-44.2068, 107.075) ccw
  line L256 (-44.2068, 107.575) -> (-38.2068, 107.575)
  arc A257 (-37.7068, 107.075) -> (-38.2068, 107.575) centre (-38.2068, 107.075) ccw
  line L257 (-37.7068, 107.075) -> (-37.7068, 93.075)
  arc A258 (-91.825, 91.575) -> (-91.325, 92.075) centre (-91.825, 92.075) ccw
  line L258 (-91.825, 91.575) -> (-104.825, 91.575)
  arc A259 (-105.325, 92.075) -> (-104.825, 91.575) centre (-104.825, 92.075) ccw
  line L259 (-105.325, 92.075) -> (-105.325, 105.075)
  arc A260 (-104.825, 105.575) -> (-105.325, 105.075) centre (-104.825, 105.075) ccw
  line L260 (-104.825, 105.575) -> (-91.825, 105.575)
  arc A261 (-91.325, 105.075) -> (-91.825, 105.575) centre (-91.825, 105.075) ccw
  line L261 (-91.325, 105.075) -> (-91.325, 92.075)
  arc A262 (-239.4625, 110.625) -> (-238.9625, 111.125) centre (-239.4625, 111.125) ccw
  line L262 (-239.4625, 110.625) -> (-252.4625, 110.625)
  arc A263 (-252.9625, 111.125) -> (-252.4625, 110.625) centre (-252.4625, 111.125) ccw
  line L263 (-252.9625, 111.125) -> (-252.9625, 124.125)
  arc A264 (-252.4625, 124.625) -> (-252.9625, 124.125) centre (-252.4625, 124.125) ccw
  line L264 (-252.4625, 124.625) -> (-239.4625, 124.625)
  arc A265 (-238.9625, 124.125) -> (-239.4625, 124.625) centre (-239.4625, 124.125) ccw
  line L265 (-238.9625, 124.125) -> (-238.9625, 111.125)
  arc A266 (-129.925, 91.575) -> (-129.425, 92.075) centre (-129.925, 92.075) ccw
  line L266 (-129.925, 91.575) -> (-142.925, 91.575)
  arc A267 (-143.425, 92.075) -> (-142.925, 91.575) centre (-142.925, 92.075) ccw
  line L267 (-143.425, 92.075) -> (-143.425, 105.075)
  arc A268 (-142.925, 105.575) -> (-143.425, 105.075) centre (-142.925, 105.075) ccw
  line L268 (-142.925, 105.575) -> (-129.925, 105.575)
  arc A269 (-129.425, 105.075) -> (-129.925, 105.575) centre (-129.925, 105.075) ccw
  line L269 (-129.425, 105.075) -> (-129.425, 92.075)
  arc A270 (-36.2688, 92.075) -> (-35.7688, 91.575) centre (-35.7688, 92.075) ccw
  line L270 (-36.2688, 92.075) -> (-36.2688, 105.075)
  arc A271 (-35.7688, 105.575) -> (-36.2688, 105.075) centre (-35.7688, 105.075) ccw
  line L271 (-35.7688, 105.575) -> (-22.7688, 105.575)
  arc A272 (-22.2688, 105.075) -> (-22.7688, 105.575) centre (-22.7688, 105.075) ccw
  line L272 (-22.2688, 105.075) -> (-22.2688, 92.075)
  arc A273 (-22.7688, 91.575) -> (-22.2688, 92.075) centre (-22.7688, 92.075) ccw
  line L273 (-22.7688, 91.575) -> (-35.7688, 91.575)
  arc A274 (-13.2438, 110.625) -> (-12.7438, 111.125) centre (-13.2438, 111.125) ccw
  line L274 (-13.2438, 110.625) -> (-26.2438, 110.625)
  arc A275 (-26.7438, 111.125) -> (-26.2438, 110.625) centre (-26.2438, 111.125) ccw
  line L275 (-26.7438, 111.125) -> (-26.7438, 124.125)
  arc A276 (-26.2438, 124.625) -> (-26.7438, 124.125) centre (-26.2438, 124.125) ccw
  line L276 (-26.2438, 124.625) -> (-13.2438, 124.625)
  arc A277 (-12.7438, 124.125) -> (-13.2438, 124.625) centre (-13.2438, 124.125) ccw
  line L277 (-12.7438, 124.125) -> (-12.7438, 111.125)
  arc A278 (-20.8308, 93.075) -> (-20.3308, 92.575) centre (-20.3308, 93.075) ccw
  line L278 (-20.8308, 93.075) -> (-20.8308, 107.075)
  arc A279 (-20.3308, 107.575) -> (-20.8308, 107.075) centre (-20.3308, 107.075) ccw
  line L279 (-20.3308, 107.575) -> (-14.3308, 107.575)
  arc A280 (-13.8308, 107.075) -> (-14.3308, 107.575) centre (-14.3308, 107.075) ccw
  line L280 (-13.8308, 107.075) -> (-13.8308, 93.075)
  arc A281 (-14.3308, 92.575) -> (-13.8308, 93.075) centre (-14.3308, 93.075) ccw
  line L281 (-14.3308, 92.575) -> (-20.3308, 92.575)
  arc A282 (-29.9125, 10.6125) -> (-29.4125, 11.1125) centre (-29.9125, 11.1125) ccw
  line L282 (-29.9125, 10.6125) -> (-42.9125, 10.6125)
  arc A283 (-43.4125, 11.1125) -> (-42.9125, 10.6125) centre (-42.9125, 11.1125) ccw
  line L283 (-43.4125, 11.1125) -> (-43.4125, 24.1125)
  arc A284 (-42.9125, 24.6125) -> (-43.4125, 24.1125) centre (-42.9125, 24.1125) ccw
  line L284 (-42.9125, 24.6125) -> (-29.9125, 24.6125)
  arc A285 (-29.4125, 24.1125) -> (-29.9125, 24.6125) centre (-29.9125, 24.1125) ccw
  line L285 (-29.4125, 24.1125) -> (-29.4125, 11.1125)
  arc A286 (-15.625, 53.475) -> (-15.125, 53.975) centre (-15.625, 53.975) ccw
  line L286 (-15.625, 53.475) -> (-28.625, 53.475)
  arc A287 (-29.125, 53.975) -> (-28.625, 53.475) centre (-28.625, 53.975) ccw
  line L287 (-29.125, 53.975) -> (-29.125, 66.975)
  arc A288 (-28.625, 67.475) -> (-29.125, 66.975) centre (-28.625, 66.975) ccw
  line L288 (-28.625, 67.475) -> (-15.625, 67.475)
  arc A289 (-15.125, 66.975) -> (-15.625, 67.475) centre (-15.625, 66.975) ccw
  line L289 (-15.125, 66.975) -> (-15.125, 53.975)
  arc A290 (-120.4, 72.525) -> (-119.9, 73.025) centre (-120.4, 73.025) ccw
  line L290 (-120.4, 72.525) -> (-133.4, 72.525)
  arc A291 (-133.9, 73.025) -> (-133.4, 72.525) centre (-133.4, 73.025) ccw
  line L291 (-133.9, 73.025) -> (-133.9, 86.025)
  arc A292 (-133.4, 86.525) -> (-133.9, 86.025) centre (-133.4, 86.025) ccw
  line L292 (-133.4, 86.525) -> (-120.4, 86.525)
  arc A293 (-119.9, 86.025) -> (-120.4, 86.525) centre (-120.4, 86.025) ccw
  line L293 (-119.9, 86.025) -> (-119.9, 73.025)
  arc A294 (-268.0375, 34.425) -> (-267.5375, 34.925) centre (-268.0375, 34.925) ccw
  line L294 (-268.0375, 34.425) -> (-281.0375, 34.425)
  arc A295 (-281.5375, 34.925) -> (-281.0375, 34.425) centre (-281.0375, 34.925) ccw
  line L295 (-281.5375, 34.925) -> (-281.5375, 47.925)
  arc A296 (-281.0375, 48.425) -> (-281.5375, 47.925) centre (-281.0375, 47.925) ccw
  line L296 (-281.0375, 48.425) -> (-268.0375, 48.425)
  arc A297 (-267.5375, 47.925) -> (-268.0375, 48.425) centre (-268.0375, 47.925) ccw
  line L297 (-267.5375, 47.925) -> (-267.5375, 34.925)
  arc A298 (-134.6875, 53.475) -> (-134.1875, 53.975) centre (-134.6875, 53.975) ccw
  line L298 (-134.6875, 53.475) -> (-147.6875, 53.475)
  arc A299 (-148.1875, 53.975) -> (-147.6875, 53.475) centre (-147.6875, 53.975) ccw
  line L299 (-148.1875, 53.975) -> (-148.1875, 66.975)
  arc A300 (-147.6875, 67.475) -> (-148.1875, 66.975) centre (-147.6875, 66.975) ccw
  line L300 (-147.6875, 67.475) -> (-134.6875, 67.475)
  arc A301 (-134.1875, 66.975) -> (-134.6875, 67.475) centre (-134.6875, 66.975) ccw
  line L301 (-134.1875, 66.975) -> (-134.1875, 53.975)
  arc A302 (-144.2125, 10.6125) -> (-143.7125, 11.1125) centre (-144.2125, 11.1125) ccw
  line L302 (-144.2125, 10.6125) -> (-157.2125, 10.6125)
  arc A303 (-157.7125, 11.1125) -> (-157.2125, 10.6125) centre (-157.2125, 11.1125) ccw
  line L303 (-157.7125, 11.1125) -> (-157.7125, 24.1125)
  arc A304 (-157.2125, 24.6125) -> (-157.7125, 24.1125) centre (-157.2125, 24.1125) ccw
  line L304 (-157.2125, 24.6125) -> (-144.2125, 24.6125)
  arc A305 (-143.7125, 24.1125) -> (-144.2125, 24.6125) centre (-144.2125, 24.1125) ccw
  line L305 (-143.7125, 24.1125) -> (-143.7125, 11.1125)
  arc A306 (-60.8688, 110.625) -> (-60.3688, 111.125) centre (-60.8688, 111.125) ccw
  line L306 (-60.8688, 110.625) -> (-73.8688, 110.625)
  arc A307 (-74.3688, 111.125) -> (-73.8688, 110.625) centre (-73.8688, 111.125) ccw
  line L307 (-74.3688, 111.125) -> (-74.3688, 124.125)
  arc A308 (-73.8688, 124.625) -> (-74.3688, 124.125) centre (-73.8688, 124.125) ccw
  line L308 (-73.8688, 124.625) -> (-60.8688, 124.625)
  arc A309 (-60.3688, 124.125) -> (-60.8688, 124.625) centre (-60.8688, 124.125) ccw
  line L309 (-60.3688, 124.125) -> (-60.3688, 111.125)
  line L310 (-281.825, 109.8375) -> (-281.825, 96.8375)
  arc A310 (-282.325, 96.3375) -> (-281.825, 96.8375) centre (-282.325, 96.8375) ccw
  line L311 (-282.325, 96.3375) -> (-295.325, 96.3375)
  arc A311 (-295.825, 96.8375) -> (-295.325, 96.3375) centre (-295.325, 96.8375) ccw
  line L312 (-295.825, 96.8375) -> (-295.825, 109.8375)
  arc A312 (-295.325, 110.3375) -> (-295.825, 109.8375) centre (-295.325, 109.8375) ccw
  line L313 (-295.325, 110.3375) -> (-282.325, 110.3375)
  arc A313 (-281.825, 109.8375) -> (-282.325, 110.3375) centre (-282.325, 109.8375) ccw
  arc A314 (-29.9125, 34.425) -> (-29.4125, 34.925) centre (-29.9125, 34.925) ccw
  line L314 (-29.9125, 34.425) -> (-42.9125, 34.425)
  arc A315 (-43.4125, 34.925) -> (-42.9125, 34.425) centre (-42.9125, 34.925) ccw
  line L315 (-43.4125, 34.925) -> (-43.4125, 47.925)
  arc A316 (-42.9125, 48.425) -> (-43.4125, 47.925) centre (-42.9125, 47.925) ccw
  line L316 (-42.9125, 48.425) -> (-29.9125, 48.425)
  arc A317 (-29.4125, 47.925) -> (-29.9125, 48.425) centre (-29.9125, 47.925) ccw
  line L317 (-29.4125, 47.925) -> (-29.4125, 34.925)
  arc A318 (-314.875, 115.8875) -> (-314.375, 115.3875) centre (-314.375, 115.8875) ccw
  line L318 (-314.875, 115.8875) -> (-314.875, 128.8875)
  arc A319 (-314.375, 129.3875) -> (-314.875, 128.8875) centre (-314.375, 128.8875) ccw
  line L319 (-314.375, 129.3875) -> (-301.375, 129.3875)
  arc A320 (-300.875, 128.8875) -> (-301.375, 129.3875) centre (-301.375, 128.8875) ccw
  line L320 (-300.875, 128.8875) -> (-300.875, 115.8875)
  arc A321 (-301.375, 115.3875) -> (-300.875, 115.8875) centre (-301.375, 115.8875) ccw
  line L321 (-301.375, 115.3875) -> (-314.375, 115.3875)
  arc A322 (-132.3063, 110.625) -> (-131.8063, 111.125) centre (-132.3063, 111.125) ccw
  line L322 (-132.3063, 110.625) -> (-145.3063, 110.625)
  arc A323 (-145.8063, 111.125) -> (-145.3063, 110.625) centre (-145.3063, 111.125) ccw
  line L323 (-145.8063, 111.125) -> (-145.8063, 124.125)
  arc A324 (-145.3063, 124.625) -> (-145.8063, 124.125) centre (-145.3063, 124.125) ccw
  line L324 (-145.3063, 124.625) -> (-132.3063, 124.625)
  arc A325 (-131.8063, 124.125) -> (-132.3063, 124.625) centre (-132.3063, 124.125) ccw
  line L325 (-131.8063, 124.125) -> (-131.8063, 111.125)
  line L326 (-86.5625, 24.1125) -> (-86.5625, 11.1125)
  arc A326 (-87.0625, 10.6125) -> (-86.5625, 11.1125) centre (-87.0625, 11.1125) ccw
  line L327 (-87.0625, 10.6125) -> (-100.0625, 10.6125)
  arc A327 (-100.5625, 11.1125) -> (-100.0625, 10.6125) centre (-100.0625, 11.1125) ccw
  line L328 (-100.5625, 11.1125) -> (-100.5625, 24.1125)
  arc A328 (-100.0625, 24.6125) -> (-100.5625, 24.1125) centre (-100.0625, 24.1125) ccw
  line L329 (-100.0625, 24.6125) -> (-87.0625, 24.6125)
  arc A329 (-86.5625, 24.1125) -> (-87.0625, 24.6125) centre (-87.0625, 24.1125) ccw
  line L330 (-86.5625, 47.925) -> (-86.5625, 34.925)
  arc A330 (-87.0625, 34.425) -> (-86.5625, 34.925) centre (-87.0625, 34.925) ccw
  line L331 (-87.0625, 34.425) -> (-100.0625, 34.425)
  arc A331 (-100.5625, 34.925) -> (-100.0625, 34.425) centre (-100.0625, 34.925) ccw
  line L332 (-100.5625, 34.925) -> (-100.5625, 47.925)
  arc A332 (-100.0625, 48.425) -> (-100.5625, 47.925) centre (-100.0625, 47.925) ccw
  line L333 (-100.0625, 48.425) -> (-87.0625, 48.425)
  arc A333 (-86.5625, 47.925) -> (-87.0625, 48.425) centre (-87.0625, 47.925) ccw
  arc A334 (-214.8625, 11.1125) -> (-214.3625, 10.6125) centre (-214.3625, 11.1125) ccw
  line L334 (-214.8625, 11.1125) -> (-214.8625, 24.1125)
  arc A335 (-214.3625, 24.6125) -> (-214.8625, 24.1125) centre (-214.3625, 24.1125) ccw
  line L335 (-214.3625, 24.6125) -> (-201.3625, 24.6125)
  arc A336 (-200.8625, 24.1125) -> (-201.3625, 24.6125) centre (-201.3625, 24.1125) ccw
  line L336 (-200.8625, 24.1125) -> (-200.8625, 11.1125)
  arc A337 (-201.3625, 10.6125) -> (-200.8625, 11.1125) centre (-201.3625, 11.1125) ccw
  line L337 (-201.3625, 10.6125) -> (-214.3625, 10.6125)
  line L338 (-281.825, 128.8875) -> (-281.825, 115.8875)
  arc A338 (-282.325, 115.3875) -> (-281.825, 115.8875) centre (-282.325, 115.8875) ccw
  line L339 (-282.325, 115.3875) -> (-295.325, 115.3875)
  arc A339 (-295.825, 115.8875) -> (-295.325, 115.3875) centre (-295.325, 115.8875) ccw
  line L340 (-295.825, 115.8875) -> (-295.825, 128.8875)
  arc A340 (-295.325, 129.3875) -> (-295.825, 128.8875) centre (-295.325, 128.8875) ccw
  line L341 (-295.325, 129.3875) -> (-282.325, 129.3875)
  arc A341 (-281.825, 128.8875) -> (-282.325, 129.3875) centre (-282.325, 128.8875) ccw
  arc A342 (-281.0943, 73.525) -> (-280.5943, 74.025) centre (-281.0943, 74.025) ccw
  line L342 (-281.0943, 73.525) -> (-287.0943, 73.525)
  arc A343 (-287.5943, 74.025) -> (-287.0943, 73.525) centre (-287.0943, 74.025) ccw
  line L343 (-287.5943, 74.025) -> (-287.5943, 88.025)
  arc A344 (-287.0943, 88.525) -> (-287.5943, 88.025) centre (-287.0943, 88.025) ccw
  line L344 (-287.0943, 88.525) -> (-281.0943, 88.525)
  arc A345 (-280.5943, 88.025) -> (-281.0943, 88.525) centre (-281.0943, 88.025) ccw
  line L345 (-280.5943, 88.025) -> (-280.5943, 74.025)
  arc A346 (-85.8063, 111.625) -> (-85.3063, 112.125) centre (-85.8063, 112.125) ccw
  line L346 (-85.8063, 111.625) -> (-91.8063, 111.625)
  arc A347 (-92.3063, 112.125) -> (-91.8063, 111.625) centre (-91.8063, 112.125) ccw
  line L347 (-92.3063, 112.125) -> (-92.3063, 126.125)
  arc A348 (-91.8063, 126.625) -> (-92.3063, 126.125) centre (-91.8063, 126.125) ccw
  line L348 (-91.8063, 126.625) -> (-85.8063, 126.625)
  arc A349 (-85.3063, 126.125) -> (-85.8063, 126.625) centre (-85.8063, 126.125) ccw
  line L349 (-85.3063, 126.125) -> (-85.3063, 112.125)
  arc A350 (-10.8625, 10.6125) -> (-10.3625, 11.1125) centre (-10.8625, 11.1125) ccw
  line L350 (-10.8625, 10.6125) -> (-23.8625, 10.6125)
  arc A351 (-24.3625, 11.1125) -> (-23.8625, 10.6125) centre (-23.8625, 11.1125) ccw
  line L351 (-24.3625, 11.1125) -> (-24.3625, 24.1125)
  arc A352 (-23.8625, 24.6125) -> (-24.3625, 24.1125) centre (-23.8625, 24.1125) ccw
  line L352 (-23.8625, 24.6125) -> (-10.8625, 24.6125)
  arc A353 (-10.3625, 24.1125) -> (-10.8625, 24.6125) centre (-10.8625, 24.1125) ccw
  line L353 (-10.3625, 24.1125) -> (-10.3625, 11.1125)
  dimension "d15" = 140
  measures "d15" distance of L0 L2